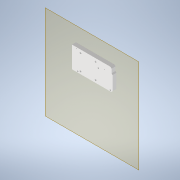
# Autodesk Inventor part: 11_Arduino_Holder
Saved by Autodesk Inventor 2021 (Build 250183000, 183)
## iProperties
Created: 2021-08-02
Part Number: 11_Arduino_Holder
Material: Generisch
Document SubType Name: Modeling
Designer: User
Density: 1 g/cm^3
Appearance: Vorgabe
Author: User
Autodesk Inventor part; units mm, degrees
ref_plane "YZ Plane" through (0, 0, 0) normal (1, 0, 0) x (0, 1, 0)
ref_plane "XZ Plane" through (0, 0, 0) normal (0, 1, 0) x (-1, 0, 0)
ref_plane "XY Plane" through (0, 0, 0) normal (0, 0, 1) x (1, 0, 0)
ref_plane "Arbeitsebene1" through (0, 0, 0) normal (0, 0, 1) x (1, 0, 0)
sketch "Skizze1" plane through (0, 0, 0) normal (0, 0, 1) x (1, 0, 0)
  circle A0 centre (19, 73.7337) radius 2 projected
  circle A1 centre (19, 33.7337) radius 2 projected
  circle A2 centre (-19, 33.7337) radius 2 projected
  circle A3 centre (-19, 73.7337) radius 2 projected
  circle A4 centre (-26.0164, 30.4697) radius 1.6 projected
  circle A5 centre (56.4536, 30.4697) radius 1.6 projected
  circle A6 centre (26.0036, 63.4597) radius 1.6 projected
  circle A7 centre (-24.7864, 78.6897) radius 1.6 construction
  circle A8 centre (-28.7864, 78.6897) radius 1.2
  circle A9 centre (26.0036, 63.4597) radius 1.5753
  circle A10 centre (56.4536, 30.4697) radius 1.5753
  circle A11 centre (-26.0164, 30.4697) radius 1.5753
  circle A12 centre (19, 33.7337) radius 2.1
  circle A13 centre (-19, 33.7337) radius 2.1
  circle A14 centre (-19, 73.7337) radius 2.1
  circle A15 centre (19, 73.7337) radius 2.1
  circle A16 centre (50.0936, 78.6897) radius 1.6 construction
  circle A17 centre (42.0936, 68.6897) radius 1.2
  line L0 (-39.0164, 27.9297) -> (57.9636, 27.9297) projected
  arc A18 (57.9636, 27.9297) -> (58.9636, 28.9297) centre (57.9636, 28.9297) ccw projected
  line L1 (58.9636, 29.1897) -> (61.5036, 31.7297) projected
  line L2 (58.9636, 28.9297) -> (58.9636, 29.1897) projected
  line L3 (61.5036, 31.7297) -> (61.5036, 65.9897) projected
  line L4 (61.5036, 65.9897) -> (58.9636, 68.5297) projected
  line L5 (58.9636, 68.5297) -> (58.9636, 78.6897) projected
  line L6 (58.9636, 78.6897) -> (56.4236, 81.2297) projected
  line L7 (56.4236, 81.2297) -> (-39.0164, 81.2297) projected
  arc A19 (-39.0164, 81.2297) -> (-40.0164, 80.2297) centre (-39.0164, 80.2297) ccw projected
  line L8 (-40.0164, 80.2297) -> (-40.0164, 72.2297) projected
  line L9 (-40.0164, 60.2297) -> (-40.0164, 40.3297) projected
  arc A20 (-40.0164, 28.9297) -> (-39.0164, 27.9297) centre (-39.0164, 28.9297) ccw projected
  line L10 (-40.0164, 31.3297) -> (-40.0164, 28.9297) projected
  line L11 (58.7921, 26.9297) -> (62.5036, 30.6413)
  line L12 (62.5036, 30.6413) -> (62.5036, 66.4039)
  line L13 (62.5036, 66.4039) -> (59.9636, 68.9439)
  line L14 (59.9636, 68.9439) -> (59.9636, 79.1039)
  line L15 (59.9636, 79.1039) -> (56.8379, 82.2297)
  line L16 (56.8379, 82.2297) -> (-41.0164, 82.2297)
  line L17 (-41.0164, 82.2297) -> (-41.0164, 26.9297)
  line L18 (-41.0164, 26.9297) -> (58.7921, 26.9297)
  point P0 (0, 0)
  dimension "d0" = 2.4
  dimension "d1" = 4
  dimension "d2" = 3.1505
  dimension "d3" = 3.1505
  dimension "d4" = 3.1505
  dimension "d5" = 0.1
  dimension "d6" = 0.1
  dimension "d7" = 0.1
  dimension "d8" = 0.1
  dimension "d9" = 2.4
  dimension "d10" = 10
  dimension "d11" = 8
  dimension "d12" = 1
  dimension "d13" = 1
  dimension "d14" = 1
  dimension "d15" = 1
  dimension "d16" = 1
  dimension "d17" = 1
  dimension "d18" = 1
  dimension "d19" = 1
  constraints: 16 end point, 9 centre point, 8 parallel, 7 coincident, 1 horizontal alignment, 1 perpendicular
  measures "d0" diameter of A8
  measures "d1" distance of A7.centre A8.centre
  measures "d2" diameter of A10
  measures "d3" diameter of A11
  measures "d4" diameter of A9
  measures "d5" radial gap between concentric circles of A1 A12
  measures "d6" radial gap between concentric circles of A2 A13
  measures "d7" radial gap between concentric circles of A0 A15
  measures "d8" radial gap between concentric circles of A3 A14
  measures "d9" diameter of A17
  measures "d10" vertical distance of A17.centre A16.centre
  measures "d11" horizontal distance of A17.centre A16.centre
  measures "d12" distance between parallel lines of L18 L0
  measures "d13" distance edge to line of A18 L11
  measures "d14" distance between parallel lines of L12 L3
  measures "d15" distance between parallel lines of L4 L13
  measures "d16" distance between parallel lines of L14 L5
  measures "d17" distance between parallel lines of L6 L15
  measures "d18" distance between parallel lines of L7 L16
  measures "d19" distance between parallel lines of L8 L17
extrude "Extrusion1" add sketch "Skizze1" along normal blind 1.6 contours A4 | A5 | A6 | A8 | A17 | L18 L17 L16 L15 L14 L13 L12 L11
sketch "Skizze2" plane through (0, 0, 1.6) normal (0, 0, 1) x (1, 0, 0)
  circle A0 centre (42.0936, 68.6897) radius 1.2 projected
  circle A1 centre (-28.7864, 78.6897) radius 1.2 projected
  circle A2 centre (56.4536, 30.4697) radius 1.5752 projected
  circle A3 centre (-26.0164, 30.4697) radius 1.5752 projected
  circle A4 centre (26.0036, 63.4597) radius 1.5752 projected
  circle A5 centre (56.4536, 30.4697) radius 3.2153
  circle A6 centre (-26.0164, 30.4697) radius 1.5752 projected
  circle A7 centre (-26.0164, 30.4697) radius 3.2153
  circle A8 centre (26.0036, 63.4597) radius 3.2153
  point P0 (0, 0)
  dimension "d22" = 1.64
  dimension "d23" = 1.64
  dimension "d24" = 1.64
  constraints: 3 centre point, 3 coincident
  measures "d22" radial gap between concentric circles of A5 A2
  measures "d23" radial gap between concentric circles of A3 A7
  measures "d24" radial gap between concentric circles of A4 A8
extrude "Extrusion2" add sketch "Skizze2" along normal blind 3.6
ref_plane "Arbeitsebene2" through (0, 0, -10) normal (-0.7604949, -0.6493439, 0) x (0, 0, 1)
chamfer "Fase1" distance 0.4 angle 45 3 edges at (-27.5916, 30.4697, 5.2) (24.4284, 63.4597, 5.2) (54.8784, 30.4697, 5.2)
sketch "Skizze4" plane through (-26.0164, 30.4697, 5.2) normal (0, 0, 1) x (1, 0, 0)
  circle A0 centre (0, 0) radius 1.5752 projected
  circle A1 centre (52.02, 32.99) radius 1.5752 projected
  circle A2 centre (82.47, 0) radius 1.5752 projected
  point P0 (26.0164, -30.4697)
  constraints: 3 coincident
sketch "Skizze3" plane through (0, 0, -10) normal (-0.7604949, -0.6493439, 0) x (0, 0, 1)
  line L0 (15.2, 41.6409) -> (15.3875, 41.9656)
  line L1 (15.3875, 41.9656) -> (15.4625, 41.9656)
  line L2 (15.4625, 41.9656) -> (15.65, 41.6409)
  line L3 (15.65, 41.6409) -> (15.725, 41.6409)
  line L4 (15.8, 41.6409) -> (15.8, 42.0306) construction
  line L5 (15.8, 42.0306) -> (15.05, 42.0306) construction
  line L6 (15.05, 42.0306) -> (15.05, 41.6409) construction
  line L7 (15.05, 41.6409) -> (15.125, 41.6409) construction
  line L8 (15.125, 41.6409) -> (15.2, 41.6409)
  line L9 (15.725, 41.6409) -> (15.8, 41.6409) construction
  line L10 (15.2, 41.6409) -> (15.65, 41.6409) construction
  line L11 (15.3875, 41.9656) -> (15.425, 42.0306) construction
  line L12 (15.4625, 41.9656) -> (15.425, 42.0306) construction
  line L13 (15.05, 40.0656) -> (15.8, 40.0656) construction
  line L14 (15.05, 41.6409) -> (15.125, 41.5109) construction
  line L15 (15.125, 41.5109) -> (15.2, 41.6409) construction
  line L16 (15.65, 41.6409) -> (15.725, 41.5109) construction
  line L17 (15.725, 41.5109) -> (15.8, 41.6409) construction
  line L18 (15.425, 41.6409) -> (15.425, 42.0306) construction
  line L19 (15.125, 41.5109) -> (15.725, 41.5109) construction
  line L20 (15.05, 40.0656) -> (15.05, 41.6409) construction
  line L21 (15.8, 40.0656) -> (15.8, 41.6409) construction
  line L22 (15.2, 41.6409) -> (15.65, 41.6409)
  line L23 (8.84, 40.0656) -> (16.96, 40.0656) projected
  line L24 (15.2, 41.6409) -> (15.2, 38.4904) projected
  dimension "d27" = 60
  dimension "d28" = 3.8
  dimension "d29" = 0.6
  dimension "d30" = 3.1505
  dimension "d31" = 0.3247
  dimension "d32" = 0.0649
  constraints: 46 end point, 11 collinear, 5 parallel, 3 midpoint, 3 perpendicular, 3 point on line, 2 coincident, 9 other
  measures "d27" angle of L0 L2
  measures "d28" diameter of L0.end L13
  measures "d29" distance of L7.end L3.end
  measures "d30" diameter of L7.end L13
  measures "d31" distance between parallel lines of L1 L10
  measures "d32" distance from line of L18.end L1
coil "Spirale1" sketch "Skizze3" operation cut axis through (-26.0164, 30.4697, 0) along (0, 0, -1) pitch 0.6 turns 9.666667 hand right
pattern_sketch "Skizzenbasierte Anordnung1" of "Spirale1" from (-26.0164, 30.4697, 5.2) copies at (26.0036, 63.4597, 5.2) at (56.4536, 30.4697, 5.2)
equation "\"d2\" = d3"
equation "\"d3\" = d36"
equation "\"d4\" = d3"
equation "\"d13\" = d12"
equation "\"d14\" = d12"
equation "\"d15\" = d12"
equation "\"d16\" = d12"
equation "\"d17\" = d12"
equation "\"d18\" = d12"
equation "\"d19\" = d12"
equation "\"d23\" = d22"
equation "\"d24\" = d22"
equation "\"d27\" = d33"
equation "\"d28\" = d34"
equation "\"d29\" = d35"
equation "\"d30\" = d36"
equation "\"d32\" = 0.125 * d37"
equation "\"d38\" = d35"
equation "\"d39\" = d25 + d20 + d38"
equation "\"d33\" = 60deg"
equation "\"d34\" = 3.8"
equation "\"d35\" = 0.6"
equation "\"d36\" = d34 - 1.0825 * d35"
equation "\"d37\" = 0.866 * d35"
equation "\"d25\" = 3.6"
equation "\"d20\" = 1.6"
